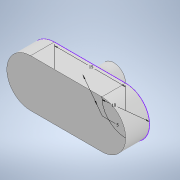
# Autodesk Inventor part: Part1
Saved by Autodesk Inventor 2022 (Build 260153000, 153)
## iProperties
Created: 2022-03-14
Part Number: Part1
Material: Generic
Document SubType Name: Modeling
Designer: br4ch
Density: 1 g/cm^3
Appearance: Default
Author: br4ch
Autodesk Inventor part; units mm, degrees
ref_plane "YZ Plane" through (0, 0, 0) normal (1, 0, 0) x (0, 1, 0)
ref_plane "XZ Plane" through (0, 0, 0) normal (0, 1, 0) x (-1, 0, 0)
ref_plane "XY Plane" through (0, 0, 0) normal (0, 0, 1) x (1, 0, 0)
sketch "Sketch1" plane through (0, 0, 0) normal (0, 0, 1) x (1, 0, 0)
  line L0 (-10, 4.2062) -> (5, 4.2062) construction
  line L1 (-10, -0.7938) -> (5, -0.7938)
  line L2 (5, 9.2062) -> (-10, 9.2062)
  arc A0 (-10, 9.2062) -> (-10, -0.7938) centre (-10, 4.2062) ccw
  arc A1 (5, -0.7938) -> (5, 9.2062) centre (5, 4.2062) ccw
  circle A2 centre (-2.5, 4.2062) radius 2.5
  point P0 (0, 0)
  dimension "d0" = 10
  dimension "d1" = 5
  dimension "d11" = 15
  constraints: 8 end point, 4 point on circle, 4 tangent, 3 centre point, 1 coincident, 1 horizontal, 1 midpoint, 1 parallel
  measures "d0" diameter of A1
  measures "d1" diameter of A2
  measures "d11" distance of L0.start L0.end
extrude "Extrusion3" add sketch "Sketch1" along normal blind 5 contours A0 L2 A1 L1 | A2
extrude "Extrusion4" add sketch "Sketch1" against normal blind 5 contours A2
body "Solid2"
